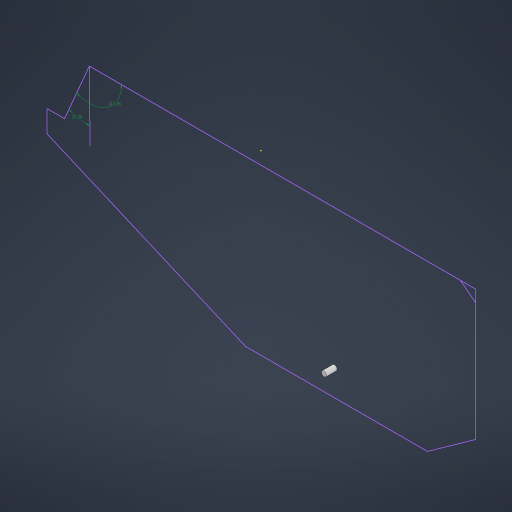
# Autodesk Inventor part: Head_CameraPanel_Bottom
Saved by Autodesk Inventor 2024 (Build 280153000, 153)
## iProperties
Created: 2025-09-16
Part Number: Head_CameraPanel_Bottom
Material: Generic
Document SubType Name: Modeling
Designer: kevin
Density: 1 g/cm^3
Appearance: Default
Author: kevin
Autodesk Inventor part; units mm, degrees
ref_plane "Work Plane1" through (0, 0.016, 0.2032) normal (0, 0, 1) x (1, 0, 0)
sketch "Sketch2" plane through (0, 0.016, 0.2032) normal (0, 0, 1) x (1, 0, 0)
  line L0 (15.65, 1.992) -> (108.35, 1.992) construction
  line L1 (15.65, 22.6862) -> (15.65, 1.992) construction
  line L2 (36.2904, 24.492) -> (15.65, 22.6862)
  line L3 (87.7096, 24.492) -> (36.2904, 24.492)
  line L4 (108.35, 22.6862) -> (87.7096, 24.492)
  line L5 (108.35, 22.6862) -> (108.35, 1.992) construction
  line L6 (51.9, 18.342) -> (72.1, 18.342)
  line L7 (72.1, 18.342) -> (72.1, 10.592)
  line L8 (72.1, 10.592) -> (51.9, 10.592)
  line L9 (51.9, 10.592) -> (51.9, 18.342)
  line L10 (72.5, 10.192) -> (72.5, 18.742)
  line L11 (72.5, 18.742) -> (51.5, 18.742)
  line L12 (51.5, 18.742) -> (51.5, 10.192)
  line L13 (51.5, 10.192) -> (72.5, 10.192)
  line L14 (124, 21.317) -> (124, 2) construction
  line L15 (124, 21.317) -> (108.35, 22.6862)
  line L16 (15.65, 22.6862) -> (0, 21.317)
  line L17 (124.5, 2) -> (124.5, 21.2813)
  line L18 (108.35, 22.6862) -> (124.5, 21.2813)
  line L19 (62, -127.908) -> (62, -8.8814) construction
  line L20 (62, -127.908) -> (193.9823, -51.708)
  line L21 (72.5, 18.742) -> (84.25, 18.742)
  line L22 (84.25, 18.742) -> (84.25, 10.2)
  line L23 (84.25, 10.2) -> (72.5, 10.2)
  line L24 (72.5, 10.2) -> (72.5, 18.742)
  line L25 (124.5, 21.2813) -> (126.4924, 21.1069)
  line L26 (84.25, 18.742) -> (115.25, 18.742)
  line L27 (115.25, 18.742) -> (115.25, 10.2)
  line L28 (115.25, 10.2) -> (84.25, 10.2)
  line L29 (84.25, 10.2) -> (84.25, 18.742)
  arc A0 (193.9823, -51.708) -> (124.5, 11.0866) centre (62, -127.908) ccw construction
  line L30 (62, -127.908) -> (62, 26.7183) construction
  line L31 (62, -127.908) -> (-69.9823, -51.708)
  line L32 (51.5, 18.742) -> (39.75, 18.742)
  line L33 (39.75, 18.742) -> (39.75, 10.2)
  line L34 (39.75, 10.2) -> (51.5, 10.2)
  line L35 (39.75, 18.742) -> (8.75, 18.742)
  line L36 (8.75, 18.742) -> (8.75, 10.2)
  line L37 (8.75, 10.2) -> (39.75, 10.2)
  circle A1 centre (62, -127.908) radius 2.1
  circle A2 centre (62, -127.908) radius 152.4 construction
  point P0 (0, -0.016)
  point P1 (124, 21.325)
  point P2 (108.35, 18.742)
  point P3 (108.35, 10.2)
  point P4 (62, 18.742)
  point P5 (62, 10.192)
  point P6 (60.1813, -126.858)
  point P7 (63.8187, -126.858)
extrude "Extrusion1" add sketch "Sketch2" along normal up to surface (8.7968 mm away) contours L31 A1 L20 | L20 A1 L31
ref_plane "Work Plane6" through (72.1, 10.608, 0) normal (1, 0, 0) x (0, 1, 0)
sketch "Sketch3" plane through (84.25, 10.216, 0.2032) normal (1, 0, 0) x (0, 0, -1)
  circle A0 centre (-4.6468, 4.267) radius 2.25 projected
  point P0 (0.2032, -10.216)
extrude "Extrusion2" [suppressed]
sketch "Sketch6" plane through (84.25, 10.216, 0.2032) normal (1, 0, 0) x (0, 0, -1)
  line L0 (-8.7968, 8.542) -> (-8.7968, 0) projected
  line L1 (0, 0) -> (-8.7968, 0) projected
  line L2 (0, 0) -> (0, 8.542) projected
  line L3 (0, 8.542) -> (-8.7968, 8.542) projected
  circle A0 centre (-4.6468, 4.267) radius 3.25
  point P0 (0.2032, -10.216)
  dimension "d10" = 6.5
  constraints: 1 centre point
  measures "d10" diameter of A0
extrude "Extrusion3" [suppressed]
ref_plane "Work Plane2" through (62, -0.5, -15.65) normal (0, -1, 0) x (-1, 0, 0)
sketch "Sketch8" plane through (62, -0.5, -15.65) normal (0, -1, 0) x (-1, 0, 0)
  arc A0 (46.35, -15.65) -> (46.35, 15.65) centre (46.35, 0) ccw projected
  arc A1 (-46.35, 15.65) -> (-46.35, -15.65) centre (-46.35, 0) ccw projected
  line L0 (-46.35, 15.65) -> (-25.7096, 15.65) projected
  line L1 (-25.7096, 15.65) -> (25.7096, 15.65) projected
  line L2 (25.7096, 15.65) -> (46.35, 15.65) projected
  line L3 (46.35, -24.65) -> (25.7096, -24.65) projected
  line L4 (25.7096, -15.8532) -> (25.7096, -24.65) projected
  line L5 (25.7096, -15.8532) -> (46.35, -15.8532) projected
  line L6 (102.4953, -24.65) -> (64.4924, -24.65) projected
  line L7 (64.4924, -15.8532) -> (64.4924, -24.65) projected
  line L8 (64.4924, -15.8532) -> (102.4953, -15.8532) projected
  line L9 (102.4953, -15.8532) -> (102.4953, -24.65) projected
  line L10 (-64.4924, -24.65) -> (-102.4516, -24.65) projected
  line L11 (-102.4516, -15.8532) -> (-102.4516, -24.65) projected
  line L12 (-102.4516, -15.8532) -> (-64.4924, -15.8532) projected
  line L13 (-64.4924, -15.8532) -> (-64.4924, -24.65) projected
  line L14 (-53.25, -15.8532) -> (-53.25, -24.65) projected
  line L15 (64.4924, -15.8532) -> (64.4924, -24.65) projected
  line L16 (46.35, -15.8532) -> (46.35, -24.65) projected
  point P0 (62, -15.65)
ref_plane "Work Plane3" through (62, 24.508, -15.65) normal (0, 1, 0) x (1, 0, 0)
ref_plane "Work Plane4" through (15.65, 2.008, -31.3) normal (0, 0, -1) x (0, 1, 0)
ref_plane "Work Plane7" through (62, 10.208, 0.2032) normal (-1, 0, 0) x (0, 0, 1)
sketch "Sketch16" plane through (0, 0.016, 0.2032) normal (0, 0, -1) x (-1, 0, 0)
  circle A0 centre (-62, -127.908) radius 2.1 projected
  circle A1 centre (-62, -127.908) radius 127
  point P0 (0, -0.016)
  dimension "d54" = 254
  constraints: 1 centre point, 1 coincident
  measures "d54" diameter of A1
extrude "Extrusion12" cut sketch "Sketch16" against normal blind 5
sketch "Sketch17" plane through (0, 0.016, 5.2032) normal (0, 0, -1) x (-1, 0, 0)
  line L0 (47.9852, -64.408) -> (-60.1813, -126.858) projected
  arc A0 (47.9852, -64.408) -> (-171.9852, -64.408) centre (-62, -127.908) ccw projected
  line L1 (-63.8187, -126.858) -> (-171.9852, -64.408) projected
  arc A1 (-60.1813, -126.858) -> (-63.8187, -126.858) centre (-62, -127.908) ccw projected
  circle A2 centre (-62, -77.108) radius 2.1
  circle A3 centre (-94.6536, -88.9929) radius 2.1
  circle A4 centre (-112.0282, -119.0867) radius 2.1
  circle A5 centre (-105.9941, -153.308) radius 2.1
  circle A6 centre (-79.3746, -175.6444) radius 2.1
  circle A7 centre (-44.6254, -175.6444) radius 2.1
  circle A8 centre (-18.0059, -153.308) radius 2.1
  circle A9 centre (-11.9718, -119.0867) radius 2.1
  circle A10 centre (-29.3464, -88.9929) radius 2.1
  point P0 (0, -0.016)
  dimension "d57" = 4.2
  dimension "d58" = 50.8
  dimension "d61" = 360
  constraints: 9 centre point, 19 other
  measures "d57" diameter of A2
  measures "d58" distance of A2.centre A0.centre
extrude "Extrusion13" [suppressed]
sketch "Sketch19" plane through (62, -127.892, 0.2032) normal (0, 0, -1) x (-1, 0, 0)
  line L0 (228.0966, 68.2385) -> (207.1624, 117.172)
  line L1 (207.1624, 117.172) -> (168.0647, 117.172)
  line L2 (228.0966, 68.2385) -> (242.9784, 68.2385)
  line L3 (242.9784, 68.2385) -> (242.9784, 49.8254)
  line L4 (242.9784, 49.8254) -> (75.3476, -21.8884)
  line L5 (75.3476, -21.8884) -> (-78.3686, -21.8884)
  line L6 (-78.3686, -21.8884) -> (-119.2307, 7.3059)
  line L7 (-119.2307, 7.3059) -> (-119.2307, 117.172)
  line L8 (-119.2307, 117.172) -> (170.5871, 117.172)
  line L9 (-106.1144, 117.172) -> (-119.2307, 107.0826)
  line L10 (207.1624, 117.172) -> (206.5762, 59.0319)
  point P0 (62, 127.892)
  dimension "d76" = 113.162
  dimension "d77" = 23.739
  constraints: 22 end point, 3 horizontal, 3 point on line, 2 perpendicular
  measures "d76" angle of L1 L0
  measures "d77" angle of L0 L10
body "Solid1"
